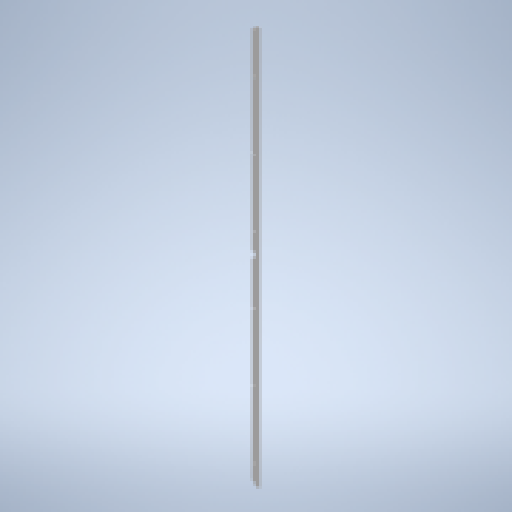
# Autodesk Inventor part: BSH 0362 stringer board 4
Saved by Autodesk Inventor 2025 (Build 290162010, 162A)
## iProperties
Created: 2024-07-23
Part Number: BSH 0362 stringer board 4
Material: 09g2s
Document SubType Name: Sheet Metal
Designer: DELL
Mass: 3894.87 g
Surface Area: 3485.79 cm^2
Volume: 496.162 cm^3
Density: 7.85 g/cm^3
Flat Pattern Width: 6.01073 cm
Flat Pattern Length: 298 cm
Flat Pattern Area: 1791.2 cm^2
Sheet Metal Rule: AISI304 3mm Die 32
Sheet Metal Width: 60,107 mm
Sheet Metal Length: 2980,000 mm
Sheet Metal Area: 179119,669 mm^2
Appearance: Default
Stock Number: БШК 0362 стрингер борт 4
Author: admin
Autodesk Inventor part; units mm, degrees
ref_plane "YZ Plane" through (0, 0, 0) normal (1, 0, 0) x (0, 1, 0)
ref_plane "XZ Plane" through (0, 0, 0) normal (0, 1, 0) x (-1, 0, 0)
ref_plane "XY Plane" through (0, 0, 0) normal (0, 0, 1) x (1, 0, 0)
sketch "Sketch6" plane through (0, 0, 0) normal (0, 1, 0) x (-1, 0, 0)
  line L0 (0, 0) -> (-60.1073, 0)
  line L1 (-60.1073, 0) -> (-60.1073, 2980)
  line L2 (-60.1073, 2980) -> (0, 2980)
  line L3 (0, 2980) -> (0, 0)
  dimension "d26" = 60.1073
  dimension "d27" = 2980
  measures "d26" distance of L1.end L2.end
  measures "d27" distance of L0.end L1.end
extrude "Plate4" add sketch "Sketch6" along normal blind 3
sketch "Sketch7" plane through (0, 0, 0) normal (0, -1, 0) x (1, 0, 0)
  line L0 (0, 2980) -> (60.1073, 2980) projected
  line L1 (0, 0) -> (0, 2980) projected
  line L2 (60.1073, 0) -> (0, 0) projected
  line L3 (60.1073, 2980) -> (60.1073, 0) projected
  line L4 (0, 145.2) -> (31.0536, 145.2)
  line L5 (31.0536, 145.2) -> (31.0536, 142)
  line L6 (31.0536, 142) -> (0, 142)
  line L7 (0, 142) -> (0, 145.2)
  point P0 (0, 142)
  point P1 (0, 200)
  point P2 (46.4173, 200)
  point P3 (0, 142)
  dimension "d29" = 31.0536
  dimension "d30" = 3.2
  dimension "d31" = 142
  constraints: 8 end point, 2 parallel, 1 horizontal, 1 perpendicular, 1 point on line
  measures "d29" distance of L5.end L6.end
  measures "d30" distance of L4.end L5.end
  measures "d31" distance between parallel lines of L2 L6
extrude "Extrusion2" cut sketch "Sketch7" against normal through all contours L4 L5 L6 L1
pattern_linear "Rectangular Pattern1" count 6 spacing 500 along (0, 0, 1) of "Extrusion2"
sketch "Sketch8" plane through (0, 0, 0) normal (0, -1, 0) x (1, 0, 0)
  line L0 (0, 1645.2) -> (0, 2142) projected
  line L1 (0, 145.2) -> (31.0536, 145.2) projected
  line L2 (31.0536, 145.2) -> (31.0536, 142) projected
  line L3 (31.0536, 142) -> (0, 142) projected
  line L4 (0, 0) -> (0, 142) projected
  line L5 (60.1073, 0) -> (0, 0) projected
  line L6 (60.1073, 2980) -> (60.1073, 0) projected
  line L7 (0, 2980) -> (60.1073, 2980) projected
  circle A0 centre (0, 1490) radius 25
  line L8 (0, 1645.2) -> (31.0536, 1645.2) projected
  line L9 (31.0536, 1645.2) -> (31.0536, 1642) projected
  line L10 (31.0536, 1642) -> (0, 1642) projected
  line L11 (0, 1145.2) -> (0, 1642) projected
  line L12 (0, 1145.2) -> (31.0536, 1145.2) projected
  line L13 (31.0536, 1145.2) -> (31.0536, 1142) projected
  line L14 (31.0536, 1142) -> (0, 1142) projected
  line L15 (0, 645.2) -> (0, 1142) projected
  line L16 (0, 645.2) -> (31.0536, 645.2) projected
  line L17 (31.0536, 645.2) -> (31.0536, 642) projected
  line L18 (31.0536, 642) -> (0, 642) projected
  line L19 (0, 145.2) -> (0, 642) projected
  line L20 (0, 2145.2) -> (31.0536, 2145.2) projected
  line L21 (31.0536, 2145.2) -> (31.0536, 2142) projected
  line L22 (31.0536, 2142) -> (0, 2142) projected
  line L23 (0, 2645.2) -> (0, 2980) projected
  line L24 (0, 2645.2) -> (31.0536, 2645.2) projected
  line L25 (31.0536, 2645.2) -> (31.0536, 2642) projected
  line L26 (31.0536, 2642) -> (0, 2642) projected
  line L27 (0, 2145.2) -> (0, 2642) projected
  dimension "d37" = 50
  dimension "d38" = 1490
  constraints: 1 centre point
  measures "d37" diameter of A0
  measures "d38" distance from line of A0.centre L5
extrude "Extrusion3" cut sketch "Sketch8" against normal through all contours L11 A0 | A0 L11
pattern_linear "Rectangular Pattern2" count 3 spacing 1480 along (0, 0, 1) of "Extrusion3" first direction both ways yes
chamfer "Corner Chamfer1" distance 6 angle 45 1 edges at (60.1073, 1.5, 2980)
chamfer "Corner Chamfer2" distance 6 angle 45 2 edges at (22.9129, 1.5, 2980) (22.9129, 1.5, 0)
sketch "Sketch10" plane through (0, 0, 0) normal (0, -1, 0) x (1, 0, 0)
  line L0 (33.0188, 174.4909) -> (18.0188, 174.4909) construction
  line L1 (18.0188, 174.4909) -> (18.0188, 374.4909) construction
  line L2 (18.0188, 374.4909) -> (33.0188, 374.4909) construction
  line L3 (33.0188, 374.4909) -> (33.0188, 174.4909) construction
  point P0 (0, 0)
  dimension "d54" = 200
  dimension "d55" = 15
  constraints: 1 vertical, 2 other
  measures "d54" distance of L0.end L1.end
  measures "d55" distance between parallel lines of L1 L3
mark "Mark2"
equation "\"d26\" = Stringer4_deep"
equation "\"d28\" = Thickness"
equation "\"BendReliefWidth\" = Thickness"
equation "\"BendReliefDepth\" = 0.5 * Thickness"
equation "\"CornerReliefSize\" = 4 * Thickness"
equation "\"MinimumRemnant\" = 2 * Thickness"
equation "\"TransitionRadius\" = BendRadius"
equation "\"JacobiRadiusSize\" = BendRadius"
equation "\"GapSize\" = Thickness"
equation "\"Stringer4_deep\" = 60.107271"
equation "\"Thickness\" = 3"
equation "\"BendRadius\" = 5"
body "Solid2"
